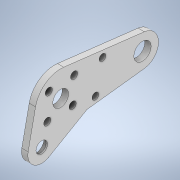
# Autodesk Inventor part: right_wall_v2
Saved by Autodesk Inventor 2020 (Build 240168000, 168)
## iProperties
Created: 2024-02-19
Part Number: right_wall_v2
Material: Типовые
Document SubType Name: Modeling
Designer: 4s
Density: 1 g/cm^3
Appearance: По умолчанию
Author: 4s
## iProperties of the stored document _3DПЕЧАТЬ.ipt
Created: 2024-03-01
Part Number: _3DПЕЧАТЬ
Material: Типовые
Document SubType Name: Modeling
Designer: 4s
Density: 1 g/cm^3
Appearance: По умолчанию
Author: 4s
Autodesk Inventor part; units mm, degrees
ref_plane "YZ Plane" through (0, 0, 0) normal (1, 0, 0) x (0, 1, 0)
ref_plane "XZ Plane" through (0, 0, 0) normal (0, 1, 0) x (-1, 0, 0)
ref_plane "XY Plane" through (0, 0, 0) normal (0, 0, 1) x (1, 0, 0)
sketch "Эскиз1" plane through (0, 0, 0) normal (1, 0, 0) x (0, 1, 0)
  circle A0 centre (35.2311, -22.6062) radius 9.3
  circle A1 centre (0, -38.8201) radius 6.1 construction
  circle A2 centre (0, 0) radius 4.85 construction
  circle A3 centre (35.8147, -49.5529) radius 3.55
  line L0 (6.0968, -38.6237) -> (4.8475, 0.1562) construction
  line L1 (-4.8475, 0.1562) -> (-6.0968, -38.6237) construction
  line L2 (0, 0) -> (0, -38.8201) construction
  circle A4 centre (0, -38.8201) radius 4.1
  circle A5 centre (0, 0) radius 2.5
  circle A6 centre (0, -38.8201) radius 15 construction
  circle A7 centre (0, 0) radius 14 construction
  circle A8 centre (0, -38.8201) radius 7.6
  circle A9 centre (0, 0) radius 7 construction
  line L3 (7.5465, -39.7207) -> (12.114, -1.4456)
  line L4 (-7.5465, -39.7207) -> (-12.114, -1.4456)
  circle A10 centre (0, 0) radius 8.8 construction
  circle A11 centre (0, 0) radius 12.2
  circle A12 centre (6.8983, -19.8347) radius 1.6
  circle A13 centre (-7.3019, -16.4524) radius 1.6
  point P0 (-7, 0)
  point P1 (-7.5465, -39.7207)
  point P2 (-12.114, -1.4456)
  dimension "d0" = 18.6
  dimension "d1" = 12.2
  dimension "d2" = 9.7
  dimension "d3" = 7.1
  dimension "d8" = 38.8201
  dimension "d13" = 38.8
  dimension "d14" = 38.8
  dimension "d23" = 8.2
  dimension "d24" = 5
  dimension "d25" = 30
  dimension "d26" = 28
  dimension "d28" = 14
  dimension "d31" = 17.6
  dimension "d32" = 3.4
  dimension "d56" = 3.5
  dimension "d58" = 3.2
  dimension "d59" = 3
  dimension "d60" = 21
  dimension "d61" = 3.2
  dimension "d62" = 3
  dimension "d63" = 18
  constraints: 12 centre point, 10 end point, 9 coincident, 4 point on circle, 4 tangent, 2 symmetric about line, 1 vertical, 8 other
  measures "d0" diameter of A0
  measures "d1" diameter of A1
  measures "d2" diameter of A2
  measures "d3" diameter of A3
  measures "d8" distance of L2.end L2.start
  measures "d13" distance of L0.start L0.end
  measures "d14" distance of L1.start L1.end
  measures "d23" diameter of A4
  measures "d24" diameter of A5
  measures "d25" diameter of A6
  measures "d26" diameter of A7
  measures "d28" diameter of A9
  measures "d31" diameter of A10
  measures "d58" diameter of A12
  measures "d59" distance from line of L3 A12.centre
  measures "d60" distance of A7.centre A12.centre
  measures "d61" diameter of A13
  measures "d62" distance from line of L4 A13.centre
  measures "d63" distance of A10.centre A13.centre
extrude "Выдавливание4" add sketch "Эскиз1" along normal blind 3 contours A8 | A8 L4 A11 L3 | A11
sketch "Эскиз4" plane through (0, 0, 0) normal (-1, 0, 0) x (0, 0, 1)
  circle A0 centre (-38.8201, 0) radius 4.1 construction
  arc A1 (-1.4456, -12.114) -> (-1.4456, 12.114) centre (0, 0) ccw construction
  line L0 (-39.7207, 7.5465) -> (-1.4456, 12.114) construction
  arc A2 (-39.7207, 7.5465) -> (-39.7207, -7.5465) centre (-38.8201, 0) ccw construction
  line L1 (-1.4456, -12.114) -> (-39.7207, -7.5465) construction
  line L2 (0, 0) -> (0, 12.2) construction
  arc A3 (-1.4456, -12.114) -> (-1.4456, 12.114) centre (0, 0) ccw construction
  line L3 (0, 0) -> (12.2, 0) construction
  circle A4 centre (5.6569, 5.6569) radius 1.7
  line L4 (5.6569, 5.6569) -> (0, 0) construction
  circle A5 centre (-6.364, 6.364) radius 1.7
  line L5 (0, 0) -> (-6.364, 6.364) construction
  circle A6 centre (-5.6569, -5.6569) radius 1.7
  circle A7 centre (6.364, -6.364) radius 1.7
  dimension "d65" = 45
  dimension "d66" = 3.4
  dimension "d67" = 3.4
  dimension "d68" = 45
  dimension "d69" = 16
  dimension "d70" = 18
  constraints: 8 end point, 4 centre point, 3 point on circle, 2 point on line, 2 symmetric about line, 1 vertical, 2 other
  measures "d65" angle of L2 L4
  measures "d66" diameter of A5
  measures "d67" diameter of A4
  measures "d68" angle of L2 L5
  measures "d69" distance of L4.start A6.centre
  measures "d70" distance of A7.centre L5.end
extrude "Выдавливание5" cut sketch "Эскиз4" against normal blind 3
sketch "Эскиз5" plane through (3, 0, 0) normal (1, 0, 0) x (0, 0, -1)
  circle A0 centre (0, 0) radius 3.75
  dimension "d38" = 7.5
  constraints: 1 centre point, 1 coincident
  measures "d38" diameter of A0
extrude "Выдавливание6" cut sketch "Эскиз5" against normal blind 3
sketch "Эскиз6" plane through (3, 0, 0) normal (1, 0, 0) x (0, 0, -1)
  circle A0 centre (0, -18) radius 2
  circle A1 centre (0, 0) radius 3.75 construction
  circle A2 centre (-5.6569, 5.6569) radius 1.7 construction
  circle A3 centre (38.8201, 0) radius 4.1 construction
  line L0 (39.7207, 7.5465) -> (1.4456, 12.114) construction
  arc A4 (1.4456, 12.114) -> (1.4456, -12.114) centre (0, 0) ccw construction
  line L1 (1.4456, -12.114) -> (39.7207, -7.5465) construction
  arc A5 (39.7207, -7.5465) -> (39.7207, 7.5465) centre (38.8201, 0) ccw construction
  line L2 (0, 0) -> (0, -26.6004) construction
  circle A6 centre (0, 0) radius 14 construction
  line L3 (-10.8605, -5.5578) -> (-3.5608, -19.8222)
  arc A7 (0, -14) -> (-3.5608, -19.8222) centre (0, -18) ccw construction
  line L4 (2.8284, -20.8284) -> (12.911, -10.7458)
  line L5 (1.4456, -12.114) -> (39.7207, -7.5465) construction
  arc A8 (2.8284, -20.8284) -> (0, -14) centre (0, -18) ccw construction
  arc A9 (-3.5608, -19.8222) -> (2.8284, -20.8284) centre (0, -18) ccw
  line L6 (-10.8605, -5.5578) -> (-10.1465, -5.5578)
  line L7 (-10.1465, -5.5578) -> (-6.8136, -9.4237)
  line L8 (-6.8136, -9.4237) -> (5.1237, -10.512)
  line L9 (5.1237, -10.512) -> (12.911, -10.7458)
  dimension "d42" = 28
  dimension "d41" = 4
  dimension "d43" = 18
  dimension "d44" = 8
  dimension "d45" = 45
  constraints: 14 end point, 7 point on circle, 5 tangent, 4 centre point, 2 coincident, 2 point on line, 1 horizontal, 1 vertical, 1 vertical alignment, 2 other
  measures "d41" diameter of A0
  measures "d43" distance of point (0, 0) A0.centre
  measures "d44" diameter of A7
  measures "d45" angle of L2 L4
extrude "Выдавливание7" [suppressed]
sketch "Эскиз7" plane through (3, 0, 0) normal (1, 0, 0) x (0, 0, -1)
  line L0 (0, 0) -> (0, -29.4139) construction
  circle A0 centre (-9, -15.5885) radius 2.75
  line L1 (-9, -15.5885) -> (0, 0) construction
  circle A1 centre (0, 0) radius 14 construction
  circle A2 centre (0, 0) radius 18 construction
  arc A3 (-5.7, -21.3042) -> (-15.4588, -14.2305) centre (-9, -15.5885) ccw construction
  circle A4 centre (0, 0) radius 3.75 construction
  circle A5 centre (-5.6569, 5.6569) radius 1.7 construction
  circle A6 centre (38.8201, 0) radius 4.1 construction
  line L2 (39.7207, 7.5465) -> (1.4456, 12.114) construction
  arc A7 (1.4456, 12.114) -> (1.4456, -12.114) centre (0, 0) ccw projected
  line L3 (1.4456, -12.114) -> (39.7207, -7.5465) projected
  arc A8 (39.7207, -7.5465) -> (39.7207, 7.5465) centre (38.8201, 0) ccw construction
  line L4 (-11.939, 2.5102) -> (-15.4588, -14.2305)
  line L5 (-5.7, -21.3042) -> (12.5035, -10.7945)
  line L6 (1.4456, -12.114) -> (39.7207, -7.5465) construction
  arc A9 (-15.4588, -14.2305) -> (-5.7, -21.3042) centre (-9, -15.5885) ccw
  circle A10 centre (-9, -15.5885) radius 4.1
  point P0 (12.5035, -10.7945)
  dimension "d48" = 5.5
  dimension "d49" = 330
  dimension "d50" = 28
  dimension "d51" = 4
  dimension "d53" = 30
  dimension "d71" = 8.2
  dimension "d76" = 2.5
  constraints: 8 end point, 5 centre point, 5 point on circle, 4 coincident, 3 tangent, 1 point on line, 1 vertical, 3 other
  measures "d48" diameter of A0
  measures "d50" diameter of A1
  measures "d53" angle of L1 L5
  measures "d71" diameter of A10
  measures "d76" radial gap between concentric circles of A10 A9
extrude "Выдавливание8" add sketch "Эскиз7" against normal up to surface (3 mm away) contours A7 L3 L5 A9 L4 | A10
extrude "Выдавливание9" cut sketch "Эскиз7" against normal blind 3 contours A10
extrude "Выдавливание10" add sketch "Эскиз7" against normal blind 0.7 contours A10
